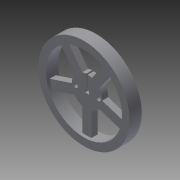
# Autodesk Inventor part: pololu_wheel_60x8
Saved by Autodesk Inventor 2014 SP1 (Build 180222100, 222)
## iProperties
Created: 2015-06-21
Part Number: pololu_wheel_60x8
Material: Générique
Document SubType Name: Modeling
Designer: astralien3000
Density: 1 g/cm^3
Appearance: Par défaut
Author: astralien3000
Autodesk Inventor part; units mm, degrees
ref_plane "YZ Plane" through (0, 0, 0) normal (1, 0, 0) x (0, 1, 0)
ref_plane "XZ Plane" through (0, 0, 0) normal (0, 1, 0) x (-1, 0, 0)
ref_plane "XY Plane" through (0, 0, 0) normal (0, 0, 1) x (1, 0, 0)
sketch "Esquisse1" plane through (0, 0, 0) normal (0, 1, 0) x (-1, 0, 0)
  circle A0 centre (0, 0) radius 30
  dimension "d0" = 60
  constraints: 1 centre point, 1 coincident
  measures "d0" diameter of A0
extrude "Extrusion1" add sketch "Esquisse1" along normal blind 8
sketch "Esquisse2" plane through (0, 8, 0) normal (0, 1, 0) x (1, 0, 0)
  circle A0 centre (0, 0) radius 30 projected
  circle A1 centre (0, 0) radius 25
  dimension "d3" = 50
  constraints: 1 centre point, 1 coincident
  measures "d3" diameter of A1
extrude "Extrusion2" cut sketch "Esquisse2" against normal blind 2 contours A1
sketch "Esquisse3" plane through (0, 0, 0) normal (0, -1, 0) x (1, 0, 0)
  circle A0 centre (0, 0) radius 30 projected
  circle A1 centre (0, 0) radius 25
  dimension "d6" = 50
  constraints: 1 centre point, 1 coincident
  measures "d6" diameter of A1
extrude "Extrusion3" cut sketch "Esquisse3" against normal blind 2 contours A1
sketch "Esquisse4" plane through (0, 6, 0) normal (0, 1, 0) x (1, 0, 0)
  circle A0 centre (0, 0) radius 25 construction
  arc A1 (3, 9.5394) -> (8.1454, 5.801) centre (0, 0) ccw construction
  line L0 (0, 0) -> (0, 25) construction
  arc A2 (3, 24.8193) -> (22.6776, 10.5228) centre (0, 0) ccw
  line L1 (0, 0) -> (23.7764, 7.7254) construction
  line L2 (3, 9.5394) -> (3, 24.8193)
  line L3 (8.1454, 5.801) -> (22.6776, 10.5228)
  arc A3 (8.1454, 5.801) -> (3, 9.5394) centre (0, 0) ccw
  arc A4 (22.6776, 10.5228) -> (3, 24.8193) centre (0, 0) ccw
  line L4 (-8.1454, 5.801) -> (-22.6776, 10.5228)
  line L5 (-3, 9.5394) -> (-3, 24.8193)
  arc A5 (-3, 9.5394) -> (-8.1454, 5.801) centre (0, 0) ccw
  arc A6 (-3, 24.8193) -> (-22.6776, 10.5228) centre (0, 0) ccw
  line L6 (-8.0342, -5.9542) -> (-17.0155, -18.3159)
  line L7 (-9.9996, 0.0947) -> (-24.5317, 4.8164)
  arc A7 (-9.9996, 0.0947) -> (-8.0342, -5.9542) centre (0, 0) ccw
  arc A8 (-24.5317, 4.8164) -> (-17.0155, -18.3159) centre (0, 0) ccw
  line L8 (3.1801, -9.4809) -> (12.1614, -21.8426)
  line L9 (-3.1801, -9.4809) -> (-12.1614, -21.8426)
  arc A9 (-3.1801, -9.4809) -> (3.1801, -9.4809) centre (0, 0) ccw
  arc A10 (-12.1614, -21.8426) -> (12.1614, -21.8426) centre (0, 0) ccw
  line L10 (9.9996, 0.0947) -> (24.5317, 4.8164)
  line L11 (8.0342, -5.9542) -> (17.0155, -18.3159)
  arc A11 (8.0342, -5.9542) -> (9.9996, 0.0947) centre (0, 0) ccw
  arc A12 (17.0155, -18.3159) -> (24.5317, 4.8164) centre (0, 0) ccw
  dimension "d9" = 20
  dimension "d10" = 72
  dimension "d11" = 3
  dimension "d12" = 3
  dimension "d15" = 360
  constraints: 30 point on circle, 24 end point, 12 centre point, 6 coincident, 2 parallel, 1 vertical, 51 other
  measures "d9" diameter of A1
  measures "d10" angle of L0 L1
  measures "d11" distance between parallel lines of L0 L2
  measures "d12" distance between parallel lines of L1 L3
extrude "Extrusion4" cut sketch "Esquisse4" against normal through all contours A4 L3 A3 L2 | L5 A5 L4 A2 | A2 L11 A11 L10 | L7 A7 L6 A2 | A2 L9 A9 L8
sketch "Esquisse5" plane through (0, 6, 0) normal (0, 1, 0) x (1, 0, 0)
  arc A0 (-3.1801, -9.4809) -> (3.1801, -9.4809) centre (0, 0) ccw construction
  arc A1 (-17.0155, -18.3159) -> (-12.1614, -21.8426) centre (0, 0) ccw projected
  arc A2 (-1.118, 1) -> (1.118, 1) centre (0, 0) ccw
  line L0 (-1.118, 1) -> (1.118, 1)
  line L1 (1.118, 1) -> (1.118, -1) construction
  line L2 (1.118, -1) -> (-1.118, -1) construction
  line L3 (-1.118, -1) -> (-1.118, 1) construction
  line L4 (-0.5, 0) -> (0.5, 0)
  line L5 (0.5, 0) -> (0.5, -9.9875)
  line L6 (0.5, -9.9875) -> (-0.5, -9.9875) construction
  line L7 (-0.5, -9.9875) -> (-0.5, 0)
  arc A3 (1.118, 1) -> (-1.118, 1) centre (0, 0) ccw
  arc A4 (0.5, -9.9875) -> (-0.5, -9.9875) centre (0, 0) ccw
  arc A5 (-0.5, -9.9875) -> (0.5, -9.9875) centre (0, 0) ccw
  dimension "d19" = 1
  dimension "d20" = 3
  dimension "d21" = 1
  constraints: 16 end point, 12 point on circle, 4 centre point, 4 parallel, 3 coincident, 2 horizontal, 2 perpendicular, 1 midpoint
  measures "d19" distance between parallel lines of L7 L5
  measures "d20" diameter of A2
  measures "d21" distance between parallel lines of L4 L0
extrude "Extrusion5" cut sketch "Esquisse5" against normal through all contours L0 A2 L5 L4 L7 | L7 L4 L5 A2 | A2 L5 A5 L7
sketch "Esquisse6" plane through (0, 6, 0) normal (0, 1, 0) x (1, 0, 0)
  arc A0 (-1.118, 1) -> (-0.5, -1.4142) centre (0, 0) ccw projected
  circle A1 centre (-7.5, 0) radius 1.5
  circle A2 centre (7.5, 0) radius 1.5
  dimension "d24" = 3
  dimension "d25" = 15
  dimension "d26" = 7.5
  dimension "d27" = 3
  constraints: 2 centre point
  measures "d24" diameter of A1
  measures "d25" distance of A2.centre A1.centre
  measures "d26" distance of A0.centre A2.centre
  measures "d27" diameter of A2
extrude "Extrusion6" cut sketch "Esquisse6" against normal through all
equation "\"d12\" = d11"
equation "\"d26\" = 0.5 * d25"
equation "\"d27\" = d24"
